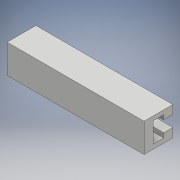
# Autodesk Inventor part: SOPORTE FINAL
Saved by Autodesk Inventor 2018.2 (Build 222227000, 227)
## iProperties
Created: 2016-05-22
Part Number: SOPORTE FINAL
Material: Genérico
Document SubType Name: Modeling
Designer: Usuario
Density: 1 g/cm^3
Appearance: Valor por defecto
Author: Usuario
Autodesk Inventor part; units mm, degrees
ref_plane "YZ Plane" through (0, 0, 0) normal (1, 0, 0) x (0, 1, 0)
ref_plane "XZ Plane" through (0, 0, 0) normal (0, 1, 0) x (-1, 0, 0)
ref_plane "XY Plane" through (0, 0, 0) normal (0, 0, 1) x (1, 0, 0)
sketch "Boceto1" plane through (0, 0, 0) normal (1, 0, 0) x (0, 1, 0)
  line L0 (0, 0) -> (0, -20.5)
  line L1 (0, -20.5) -> (10.5, -20.5)
  line L2 (10.5, -20.5) -> (10.5, -16)
  line L3 (10.5, -16) -> (20, -16)
  line L4 (0, 0) -> (10.5, 0)
  line L5 (10.5, 0) -> (10.5, -4.5)
  line L6 (10.5, -4.5) -> (20, -4.5)
  line L7 (20, 4.25) -> (-9.5, 4.25)
  line L8 (-9.5, 4.25) -> (-9.5, -25.25)
  line L9 (-9.5, -25.25) -> (20, -25.25)
  line L10 (20, 4.25) -> (20, -4.5)
  line L11 (20, -16) -> (20, -25.25)
  constraints: 24 end point, 5 perpendicular, 4 horizontal, 3 vertical
extrude "Extrusión1" add sketch "Boceto1" along normal blind 140
